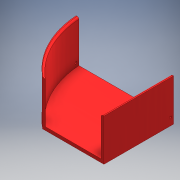
# Autodesk Inventor part: Intake Back Panel Middle
Saved by Autodesk Inventor 2016 (Build 200138000, 138)
## iProperties
Created: 2016-11-11
Part Number: Intake Back Panel Middle
Material: ABS Plastic
Document SubType Name: Modeling
Designer: paul_
Density: 1.06 g/cm^3
Appearance: Light Red
Mass: 225.869 g
Surface Area: 845.6 cm^2
Volume: 213.084 cm^3
Author: paul_
Autodesk Inventor part; units mm, degrees
ref_plane "YZ Plane" through (0, 0, 0) normal (1, 0, 0) x (0, 1, 0)
ref_plane "XZ Plane" through (0, 0, 0) normal (0, 1, 0) x (-1, 0, 0)
ref_plane "XY Plane" through (0, 0, 0) normal (0, 0, 1) x (1, 0, 0)
sketch "Sketch1" plane through (0, 0, 0) normal (0, 0, 1) x (1, 0, 0)
  line L0 (177.8, -0.9299) -> (0, -0.9299)
  line L1 (175.895, 75.2701) -> (177.8, 75.2701)
  line L2 (172.72, 5.08) -> (172.72, 72.0951)
  arc A0 (175.895, 75.2701) -> (172.72, 72.0951) centre (175.895, 72.0951) ccw
  line L3 (177.8, -0.9299) -> (177.8, 75.2701)
  line L4 (172.72, 5.08) -> (0, 5.08)
  line L5 (0, 5.08) -> (0, -0.9299)
  point P0 (172.72, 75.2701)
  dimension "d0" = 177.8
  dimension "d4" = 3.175
  dimension "d6" = 1.905
  dimension "d87" = 76.2
  constraints: 12 end point, 2 parallel, 2 point on circle, 2 tangent, 2 vertical, 1 centre point, 1 horizontal
  measures "d0" distance of L0.start L0.end
  measures "d4" radius of A0
  measures "d6" distance of L1.start L1.end
  measures "d87" distance of L1.end L0.start
extrude "Extrusion1" add sketch "Sketch1" along normal blind 127
sketch "Sketch5" plane through (0, 5.08, 0) normal (0, 1, 0) x (1, 0, 0)
  line L0 (172.72, -127) -> (71.12, -127) construction
  line L1 (0, 0) -> (0, -127) projected
  line L2 (5.08, 0) -> (0, 0)
  arc A0 (0, 0) -> (66.04, -127) centre (174.6906, 10.1687) ccw
  line L3 (71.12, -127) -> (66.04, -127)
  line L4 (172.72, -127) -> (71.12, -127)
  line L5 (0, -127) -> (177.8, -127) projected
  line L6 (172.72, -127) -> (0, -127) projected
  dimension "d99" = 5.08
  dimension "d100" = 5.08
  dimension "d134" = 101.6
  constraints: 8 end point, 2 point on circle, 1 centre point, 1 collinear, 1 horizontal, 1 point on line
  measures "d99" distance of L2.start L1.start
  measures "d100" distance of L0.end L3.end
  measures "d134" distance of L0.start L0.end
split body "Split2" sketch "Sketch5" result one side removed curves L2 A0 L3 removed pieces at (22.8484, 4.58, 104.8944)
sketch "Sketch10" plane through (172.72, 5.08, 127) normal (0, 1, 0) x (1, 0, 0)
  point P0 (-172.72, 127)
sketch "Sketch6" plane through (172.72, 5.08, 127) normal (0, 1, 0) x (1, 0, 0)
  line L0 (-106.68, 0) -> (-101.6, 0)
  line L1 (-172.72, 127) -> (0, 127) projected
  line L2 (-172.72, 127) -> (-167.64, 127)
  arc A0 (-172.72, 127) -> (-106.68, 0) centre (6.2398, 139.3887) ccw
  arc A1 (-167.64, 127) -> (-101.6, 0) centre (11.3198, 139.3887) ccw
  dimension "d135" = 5.08
  constraints: 4 end point, 4 point on circle, 2 centre point, 1 coincident, 1 horizontal, 1 point on line
  measures "d135" distance of L0.start L0.end
extrude "Extrusion3" add sketch "Sketch6" along normal blind 76.2
hole "Hole2" at (177.8, 12.5964, 5.838) direction (-1, 0, 0) diameter 4 end through all
fillet "Fillet2" radius 3.175 1 edges at (24.8837, 81.28, 70.3725)
body "Solid1"
